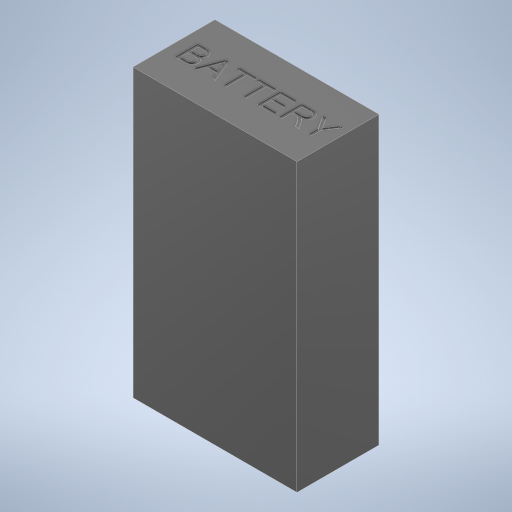
# Autodesk Inventor part: MainBattery
Saved by Autodesk Inventor 2024 (Build 280153000, 153)
## iProperties
Created: 2022-10-07
Part Number: MainBattery
Material: Generic
Document SubType Name: Modeling
Designer: Nebil
Mass: 7634 g
Surface Area: 1557.88 cm^2
Volume: 3445.03 cm^3
Density: 2.21594 g/cm^3
Appearance: Smooth - Black
Author: Nebil
Autodesk Inventor part; units mm, degrees
ref_plane "YZ Plane" through (0, 0, 0) normal (1, 0, 0) x (0, 1, 0)
ref_plane "XZ Plane" through (0, 0, 0) normal (0, 1, 0) x (-1, 0, 0)
ref_plane "XY Plane" through (0, 0, 0) normal (0, 0, 1) x (1, 0, 0)
sketch "Sketch2" plane through (0, 0, 0) normal (0, 1, 0) x (-1, 0, 0)
  line L0 (79, -39.5) -> (-79, -39.5)
  line L1 (-79, -39.5) -> (-79, 39.5)
  line L2 (-79, 39.5) -> (79, 39.5)
  line L3 (79, 39.5) -> (79, -39.5)
  line L4 (79, -39.5) -> (-79, 39.5) construction
  line L5 (-79, -39.5) -> (79, 39.5) construction
  point P0 (0, 0)
  dimension "d0" = 158
  dimension "d1" = 79
  constraints: 12 end point, 2 midpoint, 2 parallel, 1 horizontal, 1 perpendicular
  measures "d0" distance of L1.end L2.end
  measures "d1" distance of L0.end L1.end
extrude "Extrusion1" add sketch "Sketch2" along normal blind 276
sketch "Sketch3" plane through (0, 276, 0) normal (0, 1, 0) x (1, 0, 0)
  line L0 (-71.0333, 15.9179) -> (75.0167, 15.9179) construction
  line L1 (75.0167, 15.9179) -> (75.0167, -15.8321) construction
  line L2 (75.0167, -15.8321) -> (-71.0333, -15.8321) construction
  line L3 (-71.0333, -15.8321) -> (-71.0333, 15.9179) construction
  line L4 (79, -39.5) -> (79, 39.5) projected
  line L5 (79, 39.5) -> (-79, 39.5) projected
  line L6 (-79, -39.5) -> (79, -39.5) projected
  line L7 (-67.3598, -11.0696) -> (-67.3598, 11.1554)
  line L8 (-67.3598, 11.1554) -> (-59.0254, 11.1554)
  spline S0 degree 2 poles (-59.0254, 11.1554) (-56.4845, 11.1554) (-53.4014, 9.8002) (-51.6566, 7.0052) (-51.6566, 5.4636) knots 0 0 0 1 2 3 3 3
  spline S1 degree 2 poles (-51.6566, 5.4636) (-51.6566, 4.0407) (-53.1982, 1.5336) (-54.7736, 0.7544) knots 0 0 0 1 2 2 2
  spline S2 degree 2 poles (-54.7736, 0.7544) (-52.7408, 0.1615) (-50.5725, -2.6844) (-50.5725, -4.6325) knots 0 0 0 1 2 2 2
  spline S3 degree 2 poles (-50.5725, -4.6325) (-50.5725, -6.1909) (-51.8938, -8.8674) (-53.8249, -10.3242) (-56.7555, -11.0696) (-58.8899, -11.0696) knots 0 0 0 1 2 3 4 4 4
  line L9 (-58.8899, -11.0696) -> (-67.3598, -11.0696)
  line L10 (-64.4123, -8.4439) -> (-58.873, -8.4439)
  spline S4 degree 2 poles (-58.873, -8.4439) (-57.45, -8.4439) (-56.8741, -8.3423) knots 0 0 0 1 1 1
  spline S5 degree 2 poles (-56.8741, -8.3423) (-55.8577, -8.1559) (-54.4856, -7.309) (-53.6047, -5.6827) (-53.6047, -4.6155) knots 0 0 0 1 2 3 3 3
  spline S6 degree 2 poles (-53.6047, -4.6155) (-53.6047, -3.3789) (-54.9091, -1.5494) (-57.1621, -0.8041) (-59.2795, -0.8041) knots 0 0 0 1 2 3 3 3
  line L11 (-59.2795, -0.8041) -> (-64.4123, -0.8041)
  line L12 (-64.4123, -0.8041) -> (-64.4123, -8.4439)
  line L13 (-64.4123, 1.8216) -> (-59.6183, 1.8216)
  spline S7 degree 2 poles (-59.6183, 1.8216) (-57.6533, 1.8216) (-56.8063, 2.0757) knots 0 0 0 1 1 1
  spline S8 degree 2 poles (-56.8063, 2.0757) (-55.6883, 2.4145) (-54.5533, 3.956) (-54.5533, 5.1248) knots 0 0 0 1 2 2 2
  spline S9 degree 2 poles (-54.5533, 5.1248) (-54.5533, 6.2259) (-55.6205, 7.903) (-57.5856, 8.5297) (-59.9741, 8.5297) knots 0 0 0 1 2 3 3 3
  line L14 (-59.9741, 8.5297) -> (-64.4123, 8.5297)
  line L15 (-64.4123, 8.5297) -> (-64.4123, 1.8216)
  line L16 (-48.9463, -11.0696) -> (-40.4086, 11.1554)
  line L17 (-40.4086, 11.1554) -> (-37.2239, 11.1554)
  line L18 (-37.2239, 11.1554) -> (-28.1442, -11.0696)
  line L19 (-28.1442, -11.0696) -> (-31.4983, -11.0696)
  line L20 (-31.4983, -11.0696) -> (-34.0731, -4.3445)
  line L21 (-34.0731, -4.3445) -> (-43.39, -4.3445)
  line L22 (-43.39, -4.3445) -> (-45.8294, -11.0696)
  line L23 (-45.8294, -11.0696) -> (-48.9463, -11.0696)
  line L24 (-42.543, -1.956) -> (-34.9879, -1.956)
  line L25 (-34.9879, -1.956) -> (-37.3256, 4.2101)
  spline S10 degree 2 poles (-37.3256, 4.2101) (-38.3758, 7.0221) (-38.884, 8.8177) knots 0 0 0 1 1 1
  spline S11 degree 2 poles (-38.884, 8.8177) (-39.3245, 6.6833) (-40.0868, 4.5658) knots 0 0 0 1 1 1
  line L26 (-40.0868, 4.5658) -> (-42.543, -1.956)
  line L27 (-20.1486, -11.0696) -> (-20.1486, 8.5297)
  line L28 (-20.1486, 8.5297) -> (-27.4666, 8.5297)
  line L29 (-27.4666, 8.5297) -> (-27.4666, 11.1554)
  line L30 (-27.4666, 11.1554) -> (-9.8492, 11.1554)
  line L31 (-9.8492, 11.1554) -> (-9.8492, 8.5297)
  line L32 (-9.8492, 8.5297) -> (-17.2011, 8.5297)
  line L33 (-17.2011, 8.5297) -> (-17.2011, -11.0696)
  line L34 (-17.2011, -11.0696) -> (-20.1486, -11.0696)
  line L35 (-1.1761, -11.0696) -> (-1.1761, 8.5297)
  line L36 (-1.1761, 8.5297) -> (-8.4941, 8.5297)
  line L37 (-8.4941, 8.5297) -> (-8.4941, 11.1554)
  line L38 (-8.4941, 11.1554) -> (9.1233, 11.1554)
  line L39 (9.1233, 11.1554) -> (9.1233, 8.5297)
  line L40 (9.1233, 8.5297) -> (1.7715, 8.5297)
  line L41 (1.7715, 8.5297) -> (1.7715, -11.0696)
  line L42 (1.7715, -11.0696) -> (-1.1761, -11.0696)
  line L43 (12.2064, -11.0696) -> (12.2064, 11.1554)
  line L44 (12.2064, 11.1554) -> (28.2992, 11.1554)
  line L45 (28.2992, 11.1554) -> (28.2992, 8.5297)
  line L46 (28.2992, 8.5297) -> (15.1539, 8.5297)
  line L47 (15.1539, 8.5297) -> (15.1539, 1.7369)
  line L48 (15.1539, 1.7369) -> (27.4691, 1.7369)
  line L49 (27.4691, 1.7369) -> (27.4691, -0.8888)
  line L50 (27.4691, -0.8888) -> (15.1539, -0.8888)
  line L51 (15.1539, -0.8888) -> (15.1539, -8.4439)
  line L52 (15.1539, -8.4439) -> (28.8074, -8.4439)
  line L53 (28.8074, -8.4439) -> (28.8074, -11.0696)
  line L54 (28.8074, -11.0696) -> (12.2064, -11.0696)
  line L55 (32.9068, -11.0696) -> (32.9068, 11.1554)
  line L56 (32.9068, 11.1554) -> (42.7657, 11.1554)
  spline S12 degree 2 poles (42.7657, 11.1554) (45.7302, 11.1554) (48.8302, 9.9527) (50.6766, 6.9205) (50.6766, 5.091) knots 0 0 0 1 2 3 3 3
  spline S13 degree 2 poles (50.6766, 5.091) (50.6766, 2.7194) (47.6105, -0.5161) (44.4258, -0.9565) knots 0 0 0 1 2 2 2
  spline S14 degree 2 poles (44.4258, -0.9565) (45.5777, -1.5155) (46.1876, -2.0576) knots 0 0 0 1 1 1
  spline S15 degree 2 poles (46.1876, -2.0576) (47.475, -3.2434) (48.6269, -5.0221) knots 0 0 0 1 1 1
  line L57 (48.6269, -5.0221) -> (52.4722, -11.0696)
  line L58 (52.4722, -11.0696) -> (48.7963, -11.0696)
  line L59 (48.7963, -11.0696) -> (45.8488, -6.445)
  spline S16 degree 2 poles (45.8488, -6.445) (44.5614, -4.4461) (42.9013, -2.3287) (41.58, -1.4647) (40.9024, -1.2953) knots 0 0 0 1 2 3 3 3
  spline S17 degree 2 poles (40.9024, -1.2953) (40.3942, -1.1937) (39.2592, -1.1937) knots 0 0 0 1 1 1
  line L60 (39.2592, -1.1937) -> (35.8543, -1.1937)
  line L61 (35.8543, -1.1937) -> (35.8543, -11.0696)
  line L62 (35.8543, -11.0696) -> (32.9068, -11.0696)
  line L63 (35.8543, 1.3473) -> (42.1728, 1.3473)
  spline S18 degree 2 poles (42.1728, 1.3473) (44.1887, 1.3473) (46.4586, 2.1773) (47.6444, 4.0238) (47.6444, 5.091) knots 0 0 0 1 2 3 3 3
  spline S19 degree 2 poles (47.6444, 5.091) (47.6444, 6.6664) (45.3575, 8.6991) (42.8843, 8.6991) knots 0 0 0 1 2 2 2
  line L64 (42.8843, 8.6991) -> (35.8543, 8.6991)
  line L65 (35.8543, 8.6991) -> (35.8543, 1.3473)
  line L66 (61.552, -11.0696) -> (61.552, -1.6511)
  line L67 (61.552, -1.6511) -> (52.9804, 11.1554)
  line L68 (52.9804, 11.1554) -> (56.5547, 11.1554)
  line L69 (56.5547, 11.1554) -> (60.9421, 4.4473)
  spline S20 degree 2 poles (60.9421, 4.4473) (62.1787, 2.5839) (63.2121, 0.6866) knots 0 0 0 1 1 1
  spline S21 degree 2 poles (63.2121, 0.6866) (64.2115, 2.4314) (65.6344, 4.6167) knots 0 0 0 1 1 1
  line L70 (65.6344, 4.6167) -> (69.9541, 11.1554)
  line L71 (69.9541, 11.1554) -> (73.3759, 11.1554)
  line L72 (73.3759, 11.1554) -> (64.4995, -1.6511)
  line L73 (64.4995, -1.6511) -> (64.4995, -11.0696)
  line L74 (64.4995, -11.0696) -> (61.552, -11.0696)
  point P0 (0, 0)
  dimension "d4" = 146.05
  dimension "d5" = 3.9833
  dimension "d6" = 23.5821
  dimension "d8" = 31.75
  constraints: 2 other
  measures "d4" distance of L1.end L2.end
  measures "d5" distance between parallel lines of L4 L1
  measures "d6" distance between parallel lines of L5 L0
  measures "d8" distance of L2.end L0.start
emboss "Emboss1" sketch "Sketch3" operation cut depth 1.5875 direction (0, -1, 0)
equation "\"d5\" = -0.333333 * d4 + 0.333333 * d0"
equation "\"d6\" = -0.298507 * d1 + 0.298507 * d0"
body "Solid1"
